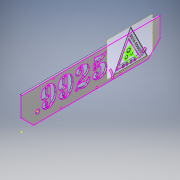
# Autodesk Inventor part: DriveTrain3.0
Saved by Autodesk Inventor 2019 (Build 230136000, 136)
## iProperties
Created: 2017-07-22
Part Number: DriveTrain3.0
Material: Aluminum 6061
Document SubType Name: Modeling
Designer: User
Density: 2.7 g/cm^3
Appearance: Aluminum - Flat
Mass: 590.045 g
Surface Area: 982.684 cm^2
Volume: 218.535 cm^3
Author: User
Autodesk Inventor part; units mm, degrees
ref_plane "YZ Plane" through (0, 0, 0) normal (1, 0, 0) x (0, 1, 0)
ref_plane "XZ Plane" through (0, 0, 0) normal (0, 1, 0) x (-1, 0, 0)
ref_plane "XY Plane" through (0, 0, 0) normal (0, 0, 1) x (1, 0, 0)
sketch "Sketch1" plane through (0, 0, 0) normal (1, 0, 0) x (0, 1, 0)
  line L0 (0, 0) -> (101.6, 0)
  line L1 (101.6, 0) -> (101.6, -444.5)
  line L2 (101.6, -444.5) -> (0, -444.5)
  line L3 (0, -444.5) -> (0, 0)
  circle A0 centre (31.75, -50.8) radius 6.3627
  circle A1 centre (31.75, -393.7) radius 6.3627
  circle A2 centre (86.2838, -165.5318) radius 1.5875
  circle A3 centre (70.2818, -165.5318) radius 1.5875
  circle A4 centre (15.3162, -278.9682) radius 1.5875
  circle A5 centre (31.3182, -278.9682) radius 1.5875
  dimension "d0" = 101.6
  dimension "d1" = 444.5
  dimension "d2" = 12.7254
  dimension "d3" = 31.75
  dimension "d4" = 50.8
  dimension "d5" = 50.8
  dimension "d22" = 165.5318
  dimension "d23" = 3.175
  dimension "d24" = 15.3162
  dimension "d25" = 3.175
  dimension "d26" = 16.002
  dimension "d27" = 165.5318
  dimension "d28" = 3.175
  dimension "d29" = 15.3162
  dimension "d30" = 165.5318
  dimension "d31" = 3.175
  dimension "d32" = 16.002
  dimension "d33" = 165.5318
  constraints: 8 end point, 6 centre point, 2 parallel, 1 horizontal, 1 perpendicular
  measures "d0" distance of L1.end L2.end
  measures "d1" distance of L0.end L1.end
  measures "d2" diameter of A0
  measures "d3" distance from line of L3 A0.centre
  measures "d4" distance from line of L0 A0.centre
  measures "d5" distance from line of L2 A1.centre
  measures "d22" distance from line of L0 A2.centre
  measures "d23" diameter of A2
  measures "d24" distance from line of L1 A2.centre
  measures "d25" diameter of A3
  measures "d26" distance of A2.centre A3.centre
  measures "d27" distance from line of L0 A3.centre
  measures "d28" diameter of A4
  measures "d29" distance from line of L3 A4.centre
  measures "d30" distance from line of L2 A4.centre
  measures "d31" diameter of A5
  measures "d32" distance of A5.centre A4.centre
  measures "d33" distance from line of L2 A5.centre
extrude "Extrusion1" add sketch "Sketch1" along normal blind 4.7625 contours L0 L1 L2 L3 | A2 | A3 | A4 | A5
chamfer "Chamfer1" distance 38.1 angle 45 1 edges at (2.3813, 0, 0)
chamfer "Chamfer2" distance 38.1 angle 45 1 edges at (2.3813, 0, -444.5)
sketch "Sketch8" plane through (4.7625, 0, 0) normal (1, 0, 0) x (0, 0, -1)
  line L0 (444.5, 38.1) -> (406.4, 0) projected
  line L1 (444.5, 38.1) -> (444.5, 101.6) projected
  line L2 (444.5, 101.6) -> (0, 101.6) projected
  line L3 (0, 101.6) -> (0, 38.1) projected
  line L4 (38.1, 0) -> (0, 38.1) projected
  line L5 (38.1, 0) -> (406.4, 0) projected
  circle A0 centre (393.7, 31.75) radius 6.3627 projected
  circle A1 centre (50.8, 31.75) radius 6.3627 projected
  point P0 (0, 0)
  point P1 (101.6, 97.155)
  point P2 (342.9, 97.155)
  point P3 (127, 4.445)
  point P4 (317.5, 4.445)
  dimension "d110" = 4.445
  dimension "d111" = 4.445
  dimension "d112" = 101.6
  dimension "d113" = 101.6
  dimension "d114" = 4.445
  dimension "d115" = 4.445
  dimension "d123" = 127
  dimension "d124" = 127
  measures "d110" distance from line of L2 point (342.9, 97.155)
  measures "d111" distance from line of L2 point (101.6, 97.155)
  measures "d112" distance from line of L3 point (101.6, 97.155)
  measures "d113" distance from line of L1 point (342.9, 97.155)
  measures "d114" distance from line of L5 point (317.5, 4.445)
  measures "d115" distance from line of L5 point (127, 4.445)
  measures "d123" distance from line of L1 point (317.5, 4.445)
  measures "d124" distance from line of L3 point (127, 4.445)
hole "Hole3" at (4.7625, 97.155, -101.6) at (4.7625, 97.155, -342.9) at (4.7625, 4.445, -127) at (4.7625, 4.445, -317.5) direction (-1, 0, 0) diameter 3.81 depth 25.4 tip angle 118
sketch "Sketch9" plane through (4.7625, 0, 0) normal (1, 0, 0) x (0, 0, -1)
  line L0 (444.5, 38.1) -> (444.5, 101.6) projected
  line L1 (38.1, 0) -> (406.4, 0) projected
  arc A0 (292.0841, 5.08) -> (284.536, 30.48) centre (241.3, 3.81) ccw construction
  arc A1 (294.6233, 5.1435) -> (286.6978, 31.8135) centre (241.3, 3.81) ccw
  arc A2 (289.5449, 5.0165) -> (282.3742, 29.1465) centre (241.3, 3.81) ccw
  arc A3 (289.5449, 5.0165) -> (294.6233, 5.1435) centre (292.0841, 5.08) ccw
  arc A4 (286.6978, 31.8135) -> (282.3742, 29.1465) centre (284.536, 30.48) ccw
  point P0 (0, 0)
  dimension "d125" = 203.2
  dimension "d126" = 3.81
  dimension "d134" = 50.8
  dimension "d135" = 5.08
  dimension "d139" = 5.08
  dimension "d140" = 25.4
  constraints: 10 point on circle, 5 centre point, 4 tangent, 1 coincident
  measures "d125" distance from line of L0 point (241.3, 3.81)
  measures "d126" distance from line of point (241.3, 3.81) L1
  measures "d134" radius of A0
  measures "d135" diameter of A4
  measures "d139" distance from line of L1 A0.start
  measures "d140" vertical distance of A0.start A0.end
hole "Hole4" at (4.7625, 3.81, -241.3) direction (-1, 0, 0) diameter 5.08 end through all
extrude "Extrusion6" cut sketch "Sketch9" against normal through all
sketch "Sketch10" plane through (4.7625, 0, 0) normal (1, 0, 0) x (0, 0, -1)
  line L0 (59.5129, 89.2474) -> (313.2288, 89.2474) construction
  line L1 (313.2288, 89.2474) -> (313.2288, 0) construction
  line L2 (313.2288, 0) -> (59.5129, 0) construction
  line L3 (59.5129, 0) -> (59.5129, 89.2474) construction
  line L4 (86.7981, 24.204) -> (86.7981, 28.8893)
  spline S0 degree 2 poles (86.7981, 28.8893) (88.2863, 29.3303) (89.8297, 30.3776) (90.381, 31.3698) knots 0 0 0 1 2 2 2
  spline S1 degree 2 poles (90.381, 31.3698) (91.5385, 33.299) (91.5385, 35.6141) knots 0 0 0 1 1 1
  line L5 (91.5385, 35.6141) -> (91.5385, 78.5538)
  spline S2 degree 2 poles (91.5385, 78.5538) (91.5385, 80.7036) (91.2629, 82.5226) (90.7668, 83.184) knots 0 0 0 1 2 2 2
  spline S3 degree 2 poles (90.7668, 83.184) (89.9951, 84.1211) (87.9005, 84.7274) knots 0 0 0 1 1 1
  line L6 (87.9005, 84.7274) -> (87.9005, 89.2474)
  spline S4 degree 2 poles (87.9005, 89.2474) (92.3653, 88.8064) (100.1926, 84.4518) (103.2243, 80.7587) knots 0 0 0 1 2 2 2
  spline S5 degree 2 poles (103.2243, 80.7587) (106.6969, 76.6797) (110.4452, 63.8364) (110.4452, 56.3398) knots 0 0 0 1 2 2 2
  spline S6 degree 2 poles (110.4452, 56.3398) (110.4452, 40.3546) (101.295, 31.0391) knots 0 0 0 1 1 1
  spline S7 degree 2 poles (101.295, 31.0391) (98.0429, 27.7869) (90.4912, 24.204) (86.7981, 24.204) knots 0 0 0 1 2 2 2
  line L7 (87.9005, 59.3715) -> (87.9005, 54.0247)
  spline S8 degree 2 poles (87.9005, 54.0247) (82.8293, 51.2687) (78.0889, 51.2687) knots 0 0 0 1 1 1
  spline S9 degree 2 poles (78.0889, 51.2687) (75.1674, 51.2687) (69.3797, 53.5286) (67.1748, 55.4579) knots 0 0 0 1 2 2 2
  spline S10 degree 2 poles (67.1748, 55.4579) (64.7495, 57.6628) (62.0485, 64.0569) (62.0485, 67.6949) knots 0 0 0 1 2 2 2
  spline S11 degree 2 poles (62.0485, 67.6949) (62.0485, 72.8763) (66.8441, 82.5777) (70.8128, 85.3338) knots 0 0 0 1 2 2 2
  spline S12 degree 2 poles (70.8128, 85.3338) (76.5455, 89.2474) (84.3727, 89.2474) knots 0 0 0 1 1 1
  line L8 (84.3727, 89.2474) -> (84.3727, 84.7274)
  spline S13 degree 2 poles (84.3727, 84.7274) (82.5537, 84.2313) (80.9552, 82.1918) (80.9552, 80.2075) knots 0 0 0 1 2 2 2
  line L9 (80.9552, 80.2075) -> (80.9552, 62.5134)
  spline S14 degree 2 poles (80.9552, 62.5134) (80.9552, 60.4188) (82.7191, 58.0486) (84.2073, 58.1037) knots 0 0 0 1 2 2 2
  spline S15 degree 2 poles (84.2073, 58.1037) (85.6405, 58.1588) (87.9005, 59.3715) knots 0 0 0 1 1 1
  line L10 (83.3254, 28.8893) -> (83.3254, 24.204)
  spline S16 degree 2 poles (83.3254, 24.204) (78.6952, 24.204) (73.9547, 26.4088) knots 0 0 0 1 1 1
  spline S17 degree 2 poles (73.9547, 26.4088) (69.986, 28.3381) (65.466, 34.4015) (65.466, 37.9292) knots 0 0 0 1 2 2 2
  spline S18 degree 2 poles (65.466, 37.9292) (65.466, 41.7878) (70.6475, 47.0243) (74.5611, 47.0243) knots 0 0 0 1 2 2 2
  spline S19 degree 2 poles (74.5611, 47.0243) (78.0337, 47.0243) (82.8844, 42.5043) (82.8844, 39.3073) knots 0 0 0 1 2 2 2
  spline S20 degree 2 poles (82.8844, 39.3073) (82.8844, 37.1024) (81.8371, 35.559) knots 0 0 0 1 1 1
  line L11 (81.8371, 35.559) -> (80.3488, 33.4644)
  spline S21 degree 2 poles (80.3488, 33.4644) (79.7425, 32.5825) (79.7425, 31.8108) knots 0 0 0 1 1 1
  spline S22 degree 2 poles (79.7425, 31.8108) (79.7425, 30.4878) (81.1757, 29.4957) knots 0 0 0 1 1 1
  spline S23 degree 2 poles (81.1757, 29.4957) (81.8922, 28.9996) (83.3254, 28.8893) knots 0 0 0 1 1 1
  line L12 (141.5337, 24.204) -> (141.5337, 28.8893)
  spline S24 degree 2 poles (141.5337, 28.8893) (143.022, 29.3303) (144.5654, 30.3776) (145.1166, 31.3698) knots 0 0 0 1 2 2 2
  spline S25 degree 2 poles (145.1166, 31.3698) (146.2742, 33.299) (146.2742, 35.6141) knots 0 0 0 1 1 1
  line L13 (146.2742, 35.6141) -> (146.2742, 78.5538)
  spline S26 degree 2 poles (146.2742, 78.5538) (146.2742, 80.7036) (145.9986, 82.5226) (145.5025, 83.184) knots 0 0 0 1 2 2 2
  spline S27 degree 2 poles (145.5025, 83.184) (144.7308, 84.1211) (142.6362, 84.7274) knots 0 0 0 1 1 1
  line L14 (142.6362, 84.7274) -> (142.6362, 89.2474)
  spline S28 degree 2 poles (142.6362, 89.2474) (147.101, 88.8064) (154.9283, 84.4518) (157.96, 80.7587) knots 0 0 0 1 2 2 2
  spline S29 degree 2 poles (157.96, 80.7587) (161.4326, 76.6797) (165.1809, 63.8364) (165.1809, 56.3398) knots 0 0 0 1 2 2 2
  spline S30 degree 2 poles (165.1809, 56.3398) (165.1809, 40.3546) (156.0307, 31.0391) knots 0 0 0 1 1 1
  spline S31 degree 2 poles (156.0307, 31.0391) (152.7785, 27.7869) (145.2269, 24.204) (141.5337, 24.204) knots 0 0 0 1 2 2 2
  line L15 (142.6362, 59.3715) -> (142.6362, 54.0247)
  spline S32 degree 2 poles (142.6362, 54.0247) (137.565, 51.2687) (132.8245, 51.2687) knots 0 0 0 1 1 1
  spline S33 degree 2 poles (132.8245, 51.2687) (129.9031, 51.2687) (124.1153, 53.5286) (121.9105, 55.4579) knots 0 0 0 1 2 2 2
  spline S34 degree 2 poles (121.9105, 55.4579) (119.4851, 57.6628) (116.7842, 64.0569) (116.7842, 67.6949) knots 0 0 0 1 2 2 2
  spline S35 degree 2 poles (116.7842, 67.6949) (116.7842, 72.8763) (121.5797, 82.5777) (125.5485, 85.3338) knots 0 0 0 1 2 2 2
  spline S36 degree 2 poles (125.5485, 85.3338) (131.2811, 89.2474) (139.1084, 89.2474) knots 0 0 0 1 1 1
  line L16 (139.1084, 89.2474) -> (139.1084, 84.7274)
  spline S37 degree 2 poles (139.1084, 84.7274) (137.2894, 84.2313) (135.6909, 82.1918) (135.6909, 80.2075) knots 0 0 0 1 2 2 2
  line L17 (135.6909, 80.2075) -> (135.6909, 62.5134)
  spline S38 degree 2 poles (135.6909, 62.5134) (135.6909, 60.4188) (137.4547, 58.0486) (138.943, 58.1037) knots 0 0 0 1 2 2 2
  spline S39 degree 2 poles (138.943, 58.1037) (140.3762, 58.1588) (142.6362, 59.3715) knots 0 0 0 1 1 1
  line L18 (138.0611, 28.8893) -> (138.0611, 24.204)
  spline S40 degree 2 poles (138.0611, 24.204) (133.4309, 24.204) (128.6904, 26.4088) knots 0 0 0 1 1 1
  spline S41 degree 2 poles (128.6904, 26.4088) (124.7217, 28.3381) (120.2017, 34.4015) (120.2017, 37.9292) knots 0 0 0 1 2 2 2
  spline S42 degree 2 poles (120.2017, 37.9292) (120.2017, 41.7878) (125.3831, 47.0243) (129.2968, 47.0243) knots 0 0 0 1 2 2 2
  spline S43 degree 2 poles (129.2968, 47.0243) (132.7694, 47.0243) (137.6201, 42.5043) (137.6201, 39.3073) knots 0 0 0 1 2 2 2
  spline S44 degree 2 poles (137.6201, 39.3073) (137.6201, 37.1024) (136.5728, 35.559) knots 0 0 0 1 1 1
  line L19 (136.5728, 35.559) -> (135.0845, 33.4644)
  spline S45 degree 2 poles (135.0845, 33.4644) (134.4782, 32.5825) (134.4782, 31.8108) knots 0 0 0 1 1 1
  spline S46 degree 2 poles (134.4782, 31.8108) (134.4782, 30.4878) (135.9113, 29.4957) knots 0 0 0 1 1 1
  spline S47 degree 2 poles (135.9113, 29.4957) (136.6279, 28.9996) (138.0611, 28.8893) knots 0 0 0 1 1 1
  line L20 (193.5685, 84.1762) -> (193.5685, 89.2474)
  line L21 (193.5685, 89.2474) -> (194.8363, 89.2474)
  spline S48 degree 2 poles (194.8363, 89.2474) (199.6869, 89.2474) (208.4513, 86.0503) (211.3727, 83.184) knots 0 0 0 1 2 2 2
  spline S49 degree 2 poles (211.3727, 83.184) (216.3336, 78.3884) (216.3336, 71.1124) knots 0 0 0 1 1 1
  spline S50 degree 2 poles (216.3336, 71.1124) (216.3336, 64.8286) (208.9474, 55.1272) (202.1123, 52.3711) knots 0 0 0 1 2 2 2
  line L22 (202.1123, 52.3711) -> (196.0489, 49.9457)
  spline S51 degree 2 poles (196.0489, 49.9457) (193.4031, 48.8984) (188.5524, 46.2526) knots 0 0 0 1 1 1
  line L23 (188.5524, 46.2526) -> (187.1744, 45.4258)
  spline S52 degree 2 poles (187.1744, 45.4258) (185.3002, 45.4258) (181.8276, 44.4336) (178.5754, 43.0555) knots 0 0 0 1 2 2 2
  spline S53 degree 2 poles (178.5754, 43.0555) (180.2842, 45.3155) (183.6466, 48.5677) (187.0641, 51.2135) knots 0 0 0 1 2 2 2
  spline S54 degree 2 poles (187.0641, 51.2135) (191.4187, 54.5759) (194.4504, 57.6076) (195.5528, 59.6471) knots 0 0 0 1 2 2 2
  spline S55 degree 2 poles (195.5528, 59.6471) (196.6001, 61.6866) (197.5923, 67.1988) (197.5923, 71.4431) knots 0 0 0 1 2 2 2
  spline S56 degree 2 poles (197.5923, 71.4431) (197.5923, 78.8845) (196.2694, 81.4753) knots 0 0 0 1 1 1
  spline S57 degree 2 poles (196.2694, 81.4753) (195.7733, 82.5226) (194.6158, 83.625) (193.5685, 84.1762) knots 0 0 0 1 2 2 2
  spline S58 degree 2 poles (215.8927, 45.6463) (216.94, 45.7014) (218.2629, 43.9375) (218.2629, 42.5043) knots 0 0 0 1 2 2 2
  spline S59 degree 2 poles (218.2629, 42.5043) (218.2629, 39.2522) (214.8454, 31.3147) (212.4751, 28.8893) knots 0 0 0 1 2 2 2
  spline S60 degree 2 poles (212.4751, 28.8893) (210.4356, 26.7947) (204.4274, 24.204) (201.7264, 24.204) knots 0 0 0 1 2 2 2
  spline S61 degree 2 poles (201.7264, 24.204) (198.4743, 24.204) (194.8363, 25.2513) knots 0 0 0 1 1 1
  line L24 (194.8363, 25.2513) -> (188.7178, 27.0703)
  spline S62 degree 2 poles (188.7178, 27.0703) (183.5363, 28.5586) (181.9929, 28.5586) knots 0 0 0 1 1 1
  spline S63 degree 2 poles (181.9929, 28.5586) (179.9534, 28.5586) (177.6935, 26.6293) knots 0 0 0 1 1 1
  spline S64 degree 2 poles (177.6935, 26.6293) (176.2603, 25.4167) (175.4886, 25.4167) knots 0 0 0 1 1 1
  spline S65 degree 2 poles (175.4886, 25.4167) (174.4413, 25.4167) (173.2837, 26.7947) (173.2837, 28.1176) knots 0 0 0 1 2 2 2
  spline S66 degree 2 poles (173.2837, 28.1176) (173.2837, 30.5981) (175.5988, 35.8346) (177.5832, 37.7639) knots 0 0 0 1 2 2 2
  spline S67 degree 2 poles (177.5832, 37.7639) (181.8276, 41.898) (189.1036, 41.898) knots 0 0 0 1 1 1
  spline S68 degree 2 poles (189.1036, 41.898) (192.5211, 41.898) (198.3089, 40.8507) knots 0 0 0 1 1 1
  spline S69 degree 2 poles (198.3089, 40.8507) (206.6874, 39.2522) (209.223, 39.2522) knots 0 0 0 1 1 1
  spline S70 degree 2 poles (209.223, 39.2522) (211.483, 39.2522) (212.5303, 40.3546) knots 0 0 0 1 1 1
  spline S71 degree 2 poles (212.5303, 40.3546) (212.9161, 40.7956) (213.3571, 41.8429) (213.6878, 43.276) knots 0 0 0 1 2 2 2
  spline S72 degree 2 poles (213.6878, 43.276) (214.1839, 45.536) (215.8927, 45.6463) knots 0 0 0 1 1 1
  line L25 (189.4343, 89.1371) -> (189.4343, 84.1762)
  spline S73 degree 2 poles (189.4343, 84.1762) (188.1114, 83.9006) (186.4578, 82.9084) (186.5129, 82.3572) knots 0 0 0 1 2 2 2
  spline S74 degree 2 poles (186.5129, 82.3572) (186.6231, 81.7509) (187.7807, 80.9792) knots 0 0 0 1 1 1
  spline S75 degree 2 poles (187.7807, 80.9792) (189.8753, 79.546) (191.7494, 76.1836) (191.7494, 73.8134) knots 0 0 0 1 2 2 2
  spline S76 degree 2 poles (191.7494, 73.8134) (191.7494, 70.2856) (186.4027, 65.1593) (182.7646, 65.1593) knots 0 0 0 1 2 2 2
  spline S77 degree 2 poles (182.7646, 65.1593) (178.7959, 65.1593) (173.5042, 70.6163) (173.5042, 74.6402) knots 0 0 0 1 2 2 2
  spline S78 degree 2 poles (173.5042, 74.6402) (173.5042, 78.4436) (178.1344, 85.0582) (182.0481, 86.9874) knots 0 0 0 1 2 2 2
  spline S79 degree 2 poles (182.0481, 86.9874) (184.5836, 88.2001) (189.4343, 89.1371) knots 0 0 0 1 1 1
  line L26 (249.8475, 58.8754) -> (249.8475, 65.6003)
  spline S80 degree 2 poles (249.8475, 65.6003) (254.6431, 65.6003) (261.1475, 64.112) (264.124, 62.3481) knots 0 0 0 1 2 2 2
  spline S81 degree 2 poles (264.124, 62.3481) (273.4947, 56.8911) (273.4947, 45.3707) knots 0 0 0 1 1 1
  spline S82 degree 2 poles (273.4947, 45.3707) (273.4947, 39.8034) (269.1952, 30.9839) (265.2816, 28.2279) knots 0 0 0 1 2 2 2
  spline S83 degree 2 poles (265.2816, 28.2279) (262.4704, 26.4088) (255.0841, 24.204) (251.4461, 24.204) knots 0 0 0 1 2 2 2
  line L27 (251.4461, 24.204) -> (249.9578, 24.204)
  line L28 (249.9578, 24.204) -> (249.9578, 29.4405)
  spline S84 degree 2 poles (249.9578, 29.4405) (251.4461, 29.8815) (253.1548, 31.3698) (253.706, 32.6376) knots 0 0 0 1 2 2 2
  spline S85 degree 2 poles (253.706, 32.6376) (254.0919, 33.4093) (254.588, 36.7166) (254.588, 38.26) knots 0 0 0 1 2 2 2
  line L29 (254.588, 38.26) -> (254.588, 50.1662)
  spline S86 degree 2 poles (254.588, 50.1662) (254.588, 54.2452) (252.6587, 57.8281) (249.8475, 58.8754) knots 0 0 0 1 2 2 2
  line L30 (233.1457, 73.8685) -> (234.4686, 89.2474)
  spline S87 degree 2 poles (234.4686, 89.2474) (236.012, 89.082) (236.2876, 89.0269) knots 0 0 0 1 1 1
  line L31 (236.2876, 89.0269) -> (245.6583, 87.8142)
  spline S88 degree 2 poles (245.6583, 87.8142) (250.6744, 87.0976) (257.5646, 87.0976) knots 0 0 0 1 1 1
  spline S89 degree 2 poles (257.5646, 87.0976) (262.2499, 87.0976) (267.9825, 88.0347) (271.1796, 89.2474) knots 0 0 0 1 2 2 2
  spline S90 degree 2 poles (271.1796, 89.2474) (270.1874, 86.0503) (267.8723, 81.9713) (265.7777, 79.8767) knots 0 0 0 1 2 2 2
  spline S91 degree 2 poles (265.7777, 79.8767) (263.5177, 77.6167) (258.1158, 74.4748) (255.4148, 73.8685) knots 0 0 0 1 2 2 2
  spline S92 degree 2 poles (255.4148, 73.8685) (251.2807, 72.9314) (244.7764, 72.9314) knots 0 0 0 1 1 1
  spline S93 degree 2 poles (244.7764, 72.9314) (238.8784, 72.9314) (233.1457, 73.8685) knots 0 0 0 1 1 1
  line L32 (245.9339, 29.4405) -> (245.9339, 24.3142)
  spline S94 degree 2 poles (245.9339, 24.3142) (241.0281, 24.645) (236.8389, 26.8498) knots 0 0 0 1 1 1
  spline S95 degree 2 poles (236.8389, 26.8498) (232.9252, 28.8893) (228.6809, 34.7873) (228.6809, 38.3151) knots 0 0 0 1 2 2 2
  spline S96 degree 2 poles (228.6809, 38.3151) (228.6809, 42.339) (233.8623, 47.7409) (237.7759, 47.7409) knots 0 0 0 1 2 2 2
  spline S97 degree 2 poles (237.7759, 47.7409) (241.0832, 47.7409) (245.989, 42.8902) (245.989, 39.5829) knots 0 0 0 1 2 2 2
  spline S98 degree 2 poles (245.989, 39.5829) (245.989, 37.7088) (244.1149, 33.8503) (242.792, 32.8581) knots 0 0 0 1 2 2 2
  spline S99 degree 2 poles (242.792, 32.8581) (241.6896, 32.0312) (241.6896, 31.5352) knots 0 0 0 1 1 1
  spline S100 degree 2 poles (241.6896, 31.5352) (241.6896, 30.7634) (243.9495, 29.661) (245.9339, 29.4405) knots 0 0 0 1 2 2 2
  line L33 (232.815, 70.2856) -> (237.1145, 69.8446)
  line L34 (237.1145, 69.8446) -> (236.2876, 60.1983)
  spline S101 degree 2 poles (236.2876, 60.1983) (239.0437, 62.4583) (243.3432, 64.7734) (245.9339, 65.4349) knots 0 0 0 1 2 2 2
  line L35 (245.9339, 65.4349) -> (245.9339, 58.8754)
  spline S102 degree 2 poles (245.9339, 58.8754) (240.973, 57.7179) (237.5554, 55.6233) knots 0 0 0 1 1 1
  spline S103 degree 2 poles (237.5554, 55.6233) (235.3506, 54.2452) (234.3033, 54.2452) knots 0 0 0 1 1 1
  spline S104 degree 2 poles (234.3033, 54.2452) (233.0355, 54.2452) (231.6023, 55.6233) (231.6023, 56.7808) knots 0 0 0 1 2 2 2
  spline S105 degree 2 poles (231.6023, 56.7808) (231.6023, 57.332) (231.6574, 58.0486) knots 0 0 0 1 1 1
  line L36 (231.6574, 58.0486) -> (232.815, 70.2856)
  point P0 (0, 0)
  constraints: 2 other
extrude "Extrusion7" cut sketch "Sketch10" against normal through all
sketch "Sketch11" plane through (4.7625, 0, 0) normal (1, 0, 0) x (0, 0, -1)
  line L0 (342.9, 86.2756) -> (381.7127, 19.05)
  line L1 (381.7127, 19.05) -> (304.0873, 19.05)
  line L2 (304.0873, 19.05) -> (342.9, 86.2756)
  line L3 (38.1, 0) -> (406.4, 0) projected
  line L4 (444.5, 101.6) -> (0, 101.6) projected
  line L5 (444.5, 38.1) -> (444.5, 101.6) projected
  point P0 (0, 0)
  point P1 (342.9, 41.4585)
  dimension "d143" = 19.05
  dimension "d144" = 19.05
  dimension "d145" = 15.3244
  dimension "d146" = 101.6
  constraints: 6 end point, 7 other
  measures "d143" distance from line of L3 L0.end
  measures "d144" distance from line of L3 L1.end
  measures "d145" distance from line of L4 L0.start
  measures "d146" distance from line of L5 L0.start
extrude "Extrusion8" cut sketch "Sketch11" against normal through all
sketch "Sketch13" plane through (4.7625, 0, 0) normal (1, 0, 0) x (0, 0, -1)
  line L0 (275.2759, 117.7277) -> (420.5521, 117.7277) construction
  line L1 (420.5521, 117.7277) -> (420.5521, 8.7705) construction
  line L2 (420.5521, 8.7705) -> (275.2759, 8.7705) construction
  line L3 (275.2759, 8.7705) -> (275.2759, 117.7277) construction
  circle A0 centre (343.7136, 55.8928) radius 7.8152
  line L4 (345.4308, 63.517) -> (345.4308, 66.3348)
  line L5 (345.4308, 66.3348) -> (342.5142, 66.3348)
  line L6 (342.5142, 66.3348) -> (342.5142, 63.6154)
  line L7 (339.1062, 62.2054) -> (336.7329, 64.4193)
  line L8 (336.7329, 64.4193) -> (334.6677, 62.2054)
  line L9 (334.6677, 62.2054) -> (337.0964, 60.051)
  line L10 (335.984, 57.0462) -> (326.0244, 57.0462)
  line L11 (324.4099, 54.2498) -> (336.0731, 54.2498)
  line L12 (337.0964, 51.7346) -> (334.9002, 49.3803)
  line L13 (334.9002, 49.3803) -> (337.0964, 47.3315)
  line L14 (337.0964, 47.3315) -> (339.1587, 49.5422)
  line L15 (342.5142, 45.7172) -> (342.5142, 48.1702)
  line L16 (342.5142, 45.7172) -> (345.4308, 45.7172)
  line L17 (345.4308, 45.7172) -> (345.4308, 48.2686)
  line L18 (348.6314, 49.8189) -> (350.7794, 47.8152)
  line L19 (350.7794, 47.8152) -> (352.8332, 50.0169)
  line L20 (352.8332, 50.0169) -> (350.5649, 52.1329)
  line L21 (351.3541, 54.2498) -> (354.2857, 54.2498)
  line L22 (354.2857, 54.2498) -> (354.2857, 57.0753)
  line L23 (354.2857, 57.0753) -> (351.4388, 57.0753)
  line L24 (350.3289, 60.0539) -> (355.0915, 65.1593)
  line L25 (353.7847, 67.4227) -> (348.5433, 62.037)
  circle A1 centre (336.3509, 40.2473) radius 6.247
  line L26 (340.1464, 45.209) -> (340.9617, 47.3315)
  line L27 (340.9617, 47.3315) -> (339.124, 48.0375)
  line L28 (339.124, 48.0375) -> (338.3986, 46.1491)
  line L29 (335.1342, 46.3746) -> (334.3485, 48.3683)
  line L30 (334.3485, 48.3683) -> (332.3547, 47.5825)
  line L31 (332.3547, 47.5825) -> (333.1349, 45.6028)
  line L32 (331.0577, 43.5649) -> (321.0105, 48.3618)
  line L33 (319.7927, 46.2526) -> (330.2717, 41.6855)
  line L34 (330.3594, 38.4792) -> (328.268, 37.6595)
  line L35 (328.268, 37.6595) -> (329.1123, 35.5051)
  line L36 (329.1123, 35.5051) -> (331.3158, 36.5497)
  line L37 (332.9158, 35.0296) -> (331.9355, 33.1442)
  line L38 (331.9355, 33.1442) -> (334.0956, 32.2028)
  line L39 (334.0956, 32.2028) -> (334.9485, 34.1598)
  line L40 (337.6193, 34.1305) -> (344.6617, 19.2749)
  line L41 (347.5317, 19.05) -> (339.9151, 35.1169)
  line L42 (341.4084, 36.5804) -> (343.4996, 35.493)
  line L43 (343.4996, 35.493) -> (344.3752, 37.5018)
  line L44 (344.3752, 37.5018) -> (342.318, 38.3984)
  line L45 (341.9482, 43.0211) -> (343.9374, 43.8007)
  line L46 (343.9374, 43.8007) -> (344.8433, 41.8899)
  line L47 (344.8433, 41.8899) -> (342.5722, 40.8132)
  circle A2 centre (352.7571, 41.9265) radius 4.874
  line L48 (354.3833, 46.5212) -> (354.6981, 48.15)
  line L49 (354.6981, 48.15) -> (352.9599, 48.4859)
  line L50 (352.9599, 48.4859) -> (352.6338, 46.7989)
  line L51 (349.0781, 45.1234) -> (347.8831, 46.5212)
  line L52 (347.8831, 46.5212) -> (349.0781, 47.5427)
  line L53 (349.0781, 47.5427) -> (350.2873, 46.1283)
  line L54 (348.0364, 43.1391) -> (346.5114, 43.4338)
  line L55 (346.5114, 43.4338) -> (346.1709, 41.6716)
  line L56 (346.1709, 41.6716) -> (347.8831, 41.9265)
  line L57 (348.4806, 39.5882) -> (347.027, 38.5878)
  line L58 (347.027, 38.5878) -> (348.0364, 37.1213)
  line L59 (348.0364, 37.1213) -> (349.4592, 38.3377)
  line L60 (351.4063, 37.2434) -> (351.254, 35.8184)
  line L61 (351.254, 35.8184) -> (353.0721, 35.6241)
  line L62 (353.0721, 35.6241) -> (353.2272, 37.0752)
  line L63 (355.4358, 37.8545) -> (371.8459, 19.05)
  line L64 (374.4256, 19.05) -> (356.7402, 39.1173)
  line L65 (357.3567, 40.3141) -> (359.0043, 40.1381)
  line L66 (359.0043, 40.1381) -> (359.1818, 41.799)
  line L67 (359.1818, 41.799) -> (357.631, 41.9647)
  line L68 (357.1564, 44.0246) -> (363.8751, 49.9457)
  line L69 (362.9066, 51.6231) -> (356.1864, 45.3899)
  line L70 (342.9, 86.2756) -> (304.0873, 19.05) projected
  line L71 (304.0873, 19.05) -> (381.7127, 19.05) projected
  line L72 (381.7127, 19.05) -> (342.9, 86.2756) projected
  line L73 (245.9339, 24.3142) -> (245.9339, 29.4405) projected
  line L74 (254.588, 50.1662) -> (254.588, 38.26) projected
  line L75 (249.9578, 29.4405) -> (249.9578, 24.204) projected
  line L76 (249.9578, 24.204) -> (251.4461, 24.204) projected
  line L77 (249.8475, 65.6003) -> (249.8475, 58.8754) projected
  line L78 (188.7178, 27.0703) -> (194.8363, 25.2513) projected
  line L79 (135.0845, 33.4644) -> (136.5728, 35.559) projected
  line L80 (138.0611, 24.204) -> (138.0611, 28.8893) projected
  line L81 (142.6362, 89.2474) -> (142.6362, 84.7274) projected
  line L82 (146.2742, 78.5538) -> (146.2742, 35.6141) projected
  line L83 (141.5337, 28.8893) -> (141.5337, 24.204) projected
  line L84 (80.9552, 62.5134) -> (80.9552, 80.2075) projected
  line L85 (84.3727, 84.7274) -> (84.3727, 89.2474) projected
  line L86 (87.9005, 54.0247) -> (87.9005, 59.3715) projected
  line L87 (87.9005, 89.2474) -> (87.9005, 84.7274) projected
  line L88 (91.5385, 78.5538) -> (91.5385, 35.6141) projected
  line L89 (86.7981, 28.8893) -> (86.7981, 24.204) projected
  line L90 (80.3488, 33.4644) -> (81.8371, 35.559) projected
  line L91 (83.3254, 24.204) -> (83.3254, 28.8893) projected
  line L92 (135.6909, 62.5134) -> (135.6909, 80.2075) projected
  line L93 (139.1084, 84.7274) -> (139.1084, 89.2474) projected
  line L94 (142.6362, 54.0247) -> (142.6362, 59.3715) projected
  line L95 (187.1744, 45.4258) -> (188.5524, 46.2526) projected
  line L96 (196.0489, 49.9457) -> (202.1123, 52.3711) projected
  line L97 (194.8363, 89.2474) -> (193.5685, 89.2474) projected
  line L98 (193.5685, 89.2474) -> (193.5685, 84.1762) projected
  line L99 (189.4343, 84.1762) -> (189.4343, 89.1371) projected
  line L100 (245.6583, 87.8142) -> (236.2876, 89.0269) projected
  line L101 (234.4686, 89.2474) -> (233.1457, 73.8685) projected
  line L102 (232.815, 70.2856) -> (231.6574, 58.0486) projected
  line L103 (245.9339, 58.8754) -> (245.9339, 65.4349) projected
  line L104 (236.2876, 60.1983) -> (237.1145, 69.8446) projected
  line L105 (237.1145, 69.8446) -> (232.815, 70.2856) projected
  arc A3 (286.6978, 31.8135) -> (282.3742, 29.1465) centre (284.536, 30.48) ccw projected
  arc A4 (289.5449, 5.0165) -> (282.3742, 29.1465) centre (241.3, 3.81) ccw projected
  arc A5 (289.5449, 5.0165) -> (294.6233, 5.1435) centre (292.0841, 5.08) ccw projected
  arc A6 (294.6233, 5.1435) -> (286.6978, 31.8135) centre (241.3, 3.81) ccw projected
  circle A7 centre (241.3, 3.81) radius 2.54 projected
  circle A8 centre (127, 4.445) radius 1.905 projected
  circle A9 centre (101.6, 97.155) radius 1.905 projected
  circle A10 centre (342.9, 97.155) radius 1.905 projected
  circle A11 centre (317.5, 4.445) radius 1.905 projected
  circle A12 centre (393.7, 31.75) radius 6.3627 projected
  circle A13 centre (50.8, 31.75) radius 6.3627 projected
  line L106 (406.4, 0) -> (444.5, 38.1) projected
  line L107 (406.4, 0) -> (38.1, 0) projected
  line L108 (0, 38.1) -> (38.1, 0) projected
  line L109 (0, 38.1) -> (0, 101.6) projected
  line L110 (0, 101.6) -> (444.5, 101.6) projected
  line L111 (444.5, 101.6) -> (444.5, 38.1) projected
  line L112 (342.9, 86.2756) -> (304.0873, 19.05) projected
  line L113 (304.0873, 19.05) -> (381.7127, 19.05) projected
  line L114 (381.7127, 19.05) -> (342.9, 86.2756) projected
  line L115 (245.9339, 24.3142) -> (245.9339, 29.4405) projected
  line L116 (254.588, 50.1662) -> (254.588, 38.26) projected
  line L117 (249.9578, 29.4405) -> (249.9578, 24.204) projected
  line L118 (249.9578, 24.204) -> (251.4461, 24.204) projected
  line L119 (249.8475, 65.6003) -> (249.8475, 58.8754) projected
  line L120 (188.7178, 27.0703) -> (194.8363, 25.2513) projected
  line L121 (135.0845, 33.4644) -> (136.5728, 35.559) projected
  line L122 (138.0611, 24.204) -> (138.0611, 28.8893) projected
  line L123 (142.6362, 89.2474) -> (142.6362, 84.7274) projected
  line L124 (146.2742, 78.5538) -> (146.2742, 35.6141) projected
  line L125 (141.5337, 28.8893) -> (141.5337, 24.204) projected
  line L126 (80.9552, 62.5134) -> (80.9552, 80.2075) projected
  line L127 (84.3727, 84.7274) -> (84.3727, 89.2474) projected
  line L128 (87.9005, 54.0247) -> (87.9005, 59.3715) projected
  line L129 (87.9005, 89.2474) -> (87.9005, 84.7274) projected
  line L130 (91.5385, 78.5538) -> (91.5385, 35.6141) projected
  line L131 (86.7981, 28.8893) -> (86.7981, 24.204) projected
  line L132 (80.3488, 33.4644) -> (81.8371, 35.559) projected
  line L133 (83.3254, 24.204) -> (83.3254, 28.8893) projected
  line L134 (135.6909, 62.5134) -> (135.6909, 80.2075) projected
  line L135 (139.1084, 84.7274) -> (139.1084, 89.2474) projected
  line L136 (142.6362, 54.0247) -> (142.6362, 59.3715) projected
  line L137 (187.1744, 45.4258) -> (188.5524, 46.2526) projected
  line L138 (196.0489, 49.9457) -> (202.1123, 52.3711) projected
  line L139 (194.8363, 89.2474) -> (193.5685, 89.2474) projected
  line L140 (193.5685, 89.2474) -> (193.5685, 84.1762) projected
  line L141 (189.4343, 84.1762) -> (189.4343, 89.1371) projected
  line L142 (245.6583, 87.8142) -> (236.2876, 89.0269) projected
  line L143 (234.4686, 89.2474) -> (233.1457, 73.8685) projected
  line L144 (232.815, 70.2856) -> (231.6574, 58.0486) projected
  line L145 (245.9339, 58.8754) -> (245.9339, 65.4349) projected
  line L146 (236.2876, 60.1983) -> (237.1145, 69.8446) projected
  line L147 (237.1145, 69.8446) -> (232.815, 70.2856) projected
  arc A14 (286.6978, 31.8135) -> (282.3742, 29.1465) centre (284.536, 30.48) ccw projected
  arc A15 (289.5449, 5.0165) -> (282.3742, 29.1465) centre (241.3, 3.81) ccw projected
  arc A16 (289.5449, 5.0165) -> (294.6233, 5.1435) centre (292.0841, 5.08) ccw projected
  arc A17 (294.6233, 5.1435) -> (286.6978, 31.8135) centre (241.3, 3.81) ccw projected
  circle A18 centre (241.3, 3.81) radius 2.54 projected
  circle A19 centre (127, 4.445) radius 1.905 projected
  circle A20 centre (101.6, 97.155) radius 1.905 projected
  circle A21 centre (342.9, 97.155) radius 1.905 projected
  circle A22 centre (317.5, 4.445) radius 1.905 projected
  circle A23 centre (393.7, 31.75) radius 6.3627 projected
  circle A24 centre (50.8, 31.75) radius 6.3627 projected
  line L148 (406.4, 0) -> (444.5, 38.1) projected
  line L149 (406.4, 0) -> (38.1, 0) projected
  line L150 (0, 38.1) -> (38.1, 0) projected
  line L151 (0, 38.1) -> (0, 101.6) projected
  line L152 (0, 101.6) -> (444.5, 101.6) projected
  line L153 (444.5, 101.6) -> (444.5, 38.1) projected
  point P0 (0, 0)
  constraints: 132 end point, 35 perpendicular, 13 point on line, 4 parallel, 3 horizontal, 2 vertical, 268 other
equation "\"d110\" = d111"
equation "\"d112\" = d113"
equation "\"d114\" = d111"
equation "\"d115\" = d111"
equation "\"d124\" = d123"
equation "\"d144\" = d143"
body "Solid1"
